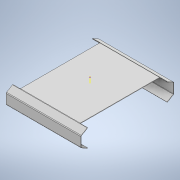
# Autodesk Inventor part: topBody
Saved by Autodesk Inventor 2020.3 (Build 243373000, 373)
## iProperties
Created: 2022-07-13
Part Number: topBody
Material: Generic
Document SubType Name: Sheet Metal
Designer: 0x6f736f646f
Density: 1 g/cm^3
Sheet Metal Rule: Default_mm
Appearance: Default
Author: 0x6f736f646f
Autodesk Inventor part; units mm, degrees
ref_plane "YZ Plane" through (0, 0, 0) normal (1, 0, 0) x (0, 1, 0)
ref_plane "XZ Plane" through (0, 0, 0) normal (0, 1, 0) x (-1, 0, 0)
ref_plane "XY Plane" through (0, 0, 0) normal (0, 0, 1) x (1, 0, 0)
sketch "Sketch1" plane through (0, 0, 0) normal (0, 1, 0) x (-1, 0, 0)
  line L0 (150, 260) -> (-150, 260)
  line L1 (-150, 260) -> (-150, -260)
  line L2 (-150, -260) -> (150, -260)
  line L3 (150, -260) -> (150, 260)
  line L4 (0, -364) -> (0, 364) projected
  line L5 (210, 0) -> (-210, 0) projected
  line L6 (150, 230) -> (-150, 230)
  line L7 (150, 190) -> (-150, 190)
  line L8 (150, 160) -> (-150, 160)
  line L9 (150, 0) -> (-150, 0)
  line L10 (150, -230) -> (-150, -230)
  line L11 (150, -190) -> (-150, -190)
  line L12 (150, -160) -> (-150, -160)
  line L13 (-120, 160) -> (-120, -160)
  line L14 (120, -160) -> (120, 160)
  line L15 (-150, 160) -> (-120, 190)
  line L16 (-120, 230) -> (-150, 260)
  line L17 (-120, 230) -> (-120, 190)
  line L18 (-150, -160) -> (-120, -190)
  line L19 (-120, -230) -> (-150, -260)
  line L20 (-120, -230) -> (-120, -190)
  line L21 (150, 160) -> (120, 190)
  line L22 (120, 230) -> (150, 260)
  line L23 (120, 230) -> (120, 190)
  line L24 (120, -230) -> (150, -260)
  line L25 (120, -230) -> (120, -190)
  line L26 (150, -160) -> (120, -190)
  point P0 (0, 0)
  point P1 (0, -260)
  point P2 (-150, 160)
  point P3 (-150, -160)
  dimension "d0" = 300
  dimension "d1" = 30
  dimension "d2" = 30
  dimension "d3" = 40
  dimension "d4" = 350
  dimension "d43" = 30
  dimension "d44" = 30
  dimension "d45" = 30
  dimension "d46" = 135
  dimension "d47" = 135
  constraints: 50 end point, 15 symmetric about line, 12 point on line, 4 parallel, 4 perpendicular, 3 midpoint, 2 vertical, 1 horizontal
  measures "d0" distance between parallel lines of L1 L3
  measures "d1" distance between parallel lines of L0 L6
  measures "d2" distance between parallel lines of L8 L7
  measures "d3" distance between parallel lines of L6 L7
  measures "d4" distance between parallel lines of L12 L7
  measures "d43" distance between parallel lines of L14 L3
  measures "d44" distance between parallel lines of L1 L13
  measures "d45" distance between parallel lines of L1 L17
  measures "d46" angle of L1 L15
  measures "d47" angle of L3 L21
extrude "Plate1" add sketch "Sketch1" along normal blind 2
fold "Fold1" angle 60 bend radius 2 thickness 2 k factor 0.44 line from (-150, 0, 230) to (150, 0, 230) line at bend centre moving side (0, 0, 1) folds toward (0, -1, 0)
fold "Fold2" angle 60 bend radius 2 thickness 2 k factor 0.44 line from (-150, 0, 190) to (150, 0, 190) line at bend centre moving side (0, 0, 1) folds toward (0, -1, 0)
fold "Fold3" angle 30 bend radius 2 thickness 2 k factor 0.44 line from (-150, 0, 160) to (150, 0, 160) line at bend centre moving side (0, 0, 1) folds toward (0, -1, 0)
fold "Fold4" angle 60 bend radius 2 thickness 2 k factor 0.44 line from (-150, 0, -230) to (150, 0, -230) line at bend centre moving side (0, 0, -1) folds toward (0, -1, 0)
fold "Fold5" angle 60 bend radius 2 thickness 2 k factor 0.44 line from (-150, 0, -190) to (150, 0, -190) line at bend centre moving side (0, 0, -1) folds toward (0, -1, 0)
fold "Fold6" angle 30 bend radius 2 thickness 2 k factor 0.44 line from (-150, 0, -160) to (150, 0, -160) line at bend centre moving side (0, 0, -1) folds toward (0, -1, 0)
sketch "Sketch2" plane through (0, 0, 0) normal (1, 0, 0) x (0, 1, 0)
  line L0 (-4.3079, 0) -> (25.8474, 0) projected
  point P0 (0, 0)
  point P1 (21.5395, 0)
  constraints: 1 point on line
extrude "Extrusion1" cut sketch "Sketch1" against normal mid plane 10 contours L3 L5 L14 L8 | L3 L12 L14 L5 | L8 L13 L5 L1 | L5 L13 L12 L1
sketch "Sketch3" plane through (-150, 1.4641, 161.246) normal (0, 0.8660254, 0.5) x (1, 0, 0)
  line L0 (300, 1.3112) -> (270, 1.3112) projected
  line L1 (300, -27.7381) -> (300, -31.2022) projected
  line L2 (270, 1.3112) -> (300, -27.7381)
  point P0 (150, 138.9111)
  constraints: 2 end point
equation "\"d5\" = Thickness"
equation "\"d6\" = BendReliefWidth"
equation "\"d7\" = BendReliefDepth"
equation "\"d8\" = MinimumRemnant"
equation "\"d9\" = TransitionRadius"
equation "\"d11\" = BendRadius"
equation "\"d12\" = BendReliefWidth"
equation "\"d13\" = BendReliefDepth"
equation "\"d14\" = MinimumRemnant"
equation "\"d15\" = TransitionRadius"
equation "\"d17\" = BendRadius"
equation "\"d18\" = BendReliefWidth"
equation "\"d19\" = BendReliefDepth"
equation "\"d20\" = MinimumRemnant"
equation "\"d21\" = TransitionRadius"
equation "\"d23\" = BendRadius"
equation "\"d24\" = BendReliefWidth"
equation "\"d25\" = BendReliefDepth"
equation "\"d26\" = MinimumRemnant"
equation "\"d27\" = TransitionRadius"
equation "\"d29\" = BendRadius"
equation "\"d30\" = BendReliefWidth"
equation "\"d31\" = BendReliefDepth"
equation "\"d32\" = MinimumRemnant"
equation "\"d33\" = TransitionRadius"
equation "\"d35\" = BendRadius"
equation "\"d36\" = BendReliefWidth"
equation "\"d37\" = BendReliefDepth"
equation "\"d38\" = MinimumRemnant"
equation "\"d39\" = TransitionRadius"
equation "\"d41\" = BendRadius"
equation "\"BendRadius\" = Thickness"
equation "\"BendReliefWidth\" = Thickness"
equation "\"BendReliefDepth\" = 0.5 * Thickness"
equation "\"CornerReliefSize\" = 4 * Thickness"
equation "\"MinimumRemnant\" = 2 * Thickness"
equation "\"TransitionRadius\" = BendRadius"
equation "\"JacobiRadiusSize\" = BendRadius"
equation "\"GapSize\" = Thickness"
equation "\"Thickness\" = 2"
body "Solid1"
